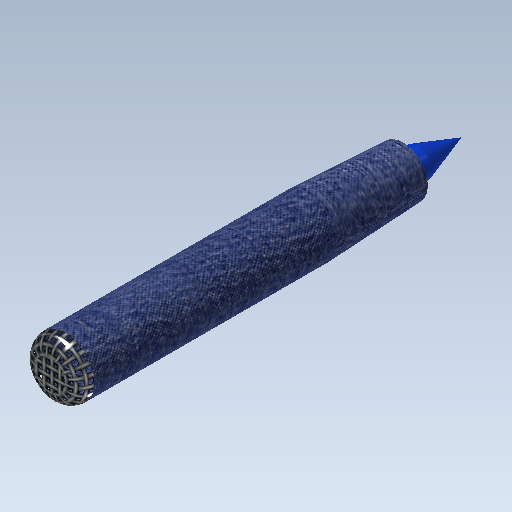
# Autodesk Inventor part: Pen
Saved by Autodesk Inventor 2021.3 (Build 253353000, 353)
## iProperties
Created: 2021-06-01
Part Number: Pen
Material: Generic
Document SubType Name: Modeling
Designer: vivek
Density: 1 g/cm^3
Appearance: Expanded Metal 04
Author: vivek
Autodesk Inventor part; units mm, degrees
ref_plane "YZ Plane" through (0, 0, 0) normal (1, 0, 0) x (0, 1, 0)
ref_plane "XZ Plane" through (0, 0, 0) normal (0, 1, 0) x (-1, 0, 0)
ref_plane "XY Plane" through (0, 0, 0) normal (0, 0, 1) x (1, 0, 0)
sketch "Sketch1" plane through (0, 0, 0) normal (0, 0, 1) x (1, 0, 0)
  circle A0 centre (0, 0) radius 10
  dimension "d0" = 20
  constraints: 1 centre point, 1 coincident
  measures "d0" diameter of A0
extrude "Extrusion1" add sketch "Sketch1" along normal blind 120
sketch "Sketch2" plane through (0, 0, 0) normal (0, 0, -1) x (-1, 0, 0)
  circle A0 centre (0, 0) radius 10 projected
  circle A1 centre (0, 0) radius 5
  dimension "d3" = 10
  constraints: 1 centre point, 1 coincident
  measures "d3" diameter of A1
extrude "Extrusion2" add sketch "Sketch2" along normal blind 20 contours A1
chamfer "Chamfer1" distance 5 distance2 15 1 edges at (5, 0, -20) measured on face at (0.591, 1.5584, -20)
chamfer "Chamfer2" distance 1.5 distance2 32.75 1 edges at (-10, 0, 0) measured on face at (8.188, -1.1966, 0)
fillet "Fillet1" radius 5 1 edges at (-10, 0, 120)
body "Solid1"
